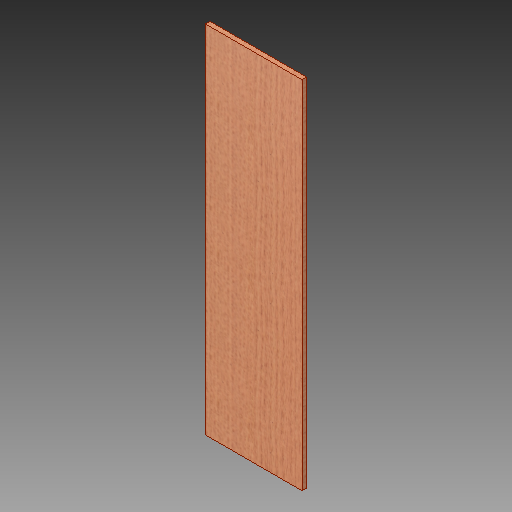
# Autodesk Inventor part: GBX_006.1-backplate_lo
Saved by Autodesk Inventor 2019 (Build 230136000, 136)
## iProperties
Created: 2019-08-15
Part Number: GBX_006.1-backplate_lo
Material: Generic
Document SubType Name: Modeling
Designer: Rene
Density: 1 g/cm^3
Appearance: Red Oak - Natural Low Gloss
Author: Rene
Autodesk Inventor part; units mm, degrees
ref_plane "YZ Plane" through (0, 0, 0) normal (1, 0, 0) x (0, 1, 0)
ref_plane "XZ Plane" through (0, 0, 0) normal (0, 1, 0) x (-1, 0, 0)
ref_plane "XY Plane" through (0, 0, 0) normal (0, 0, 1) x (1, 0, 0)
sketch "Sketch1" plane through (0, 0, 0) normal (0, 0, 1) x (1, 0, 0)
  line L0 (95, -350) -> (-95, -350)
  line L1 (-95, -350) -> (-95, 350)
  line L2 (-95, 350) -> (95, 350)
  line L3 (95, 350) -> (95, -350)
  line L4 (95, -350) -> (-95, 350) construction
  line L5 (-95, -350) -> (95, 350) construction
  point P0 (0, 0)
  dimension "d0" = 700
  dimension "d1" = 190
  constraints: 12 end point, 2 midpoint, 2 parallel, 1 horizontal, 1 perpendicular
  measures "d0" distance of L0.end L1.end
  measures "d1" distance of L1.end L2.end
extrude "Extrusion1" add sketch "Sketch1" along normal blind 9
body "Solid1"
